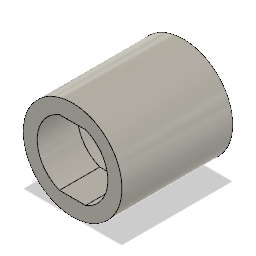
Nikon Labophot - Epifluorescence module adapter v3 (Autodesk Fusion 360 design; units mm, degrees)
Autodesk Fusion 360 part; units mm, degrees
note: some values were not read from the file. Set by a fixed rule: which sketch regions a step uses.
sketch "Sketch1" plane through (0, 0, 0) normal (0, 0, 1) x (1, 0, 0)
  circle A0 centre (0, 0) radius 22.5
  circle A1 centre (0, 0) radius 24.5
  dimension "d1" = 45
  dimension "d2" = 49
  measures "d1" diameter of A0
  measures "d2" diameter of A1
extrude "Extrude1" add sketch "Sketch1" against normal blind 35
sketch "Sketch2" plane through (0, 0, 0) normal (0, 0, 1) x (1, 0, 0)
  circle A0 centre (0, 0) radius 22.5
  circle A1 centre (0, 0) radius 24.5
  circle A2 centre (0, 0) radius 15
  circle A3 centre (0, 0) radius 17.5
  circle A4 centre (0, 0) radius 20
  line L0 (9.6825, 17.5) -> (-9.6825, 17.5)
  line L1 (-9.6825, -17.5) -> (9.6825, -17.5)
  line L2 (-11.6592, 16.25) -> (11.6592, 16.25)
  line L3 (-13.2288, 15) -> (13.2288, 15)
  line L4 (-13.2288, -15) -> (13.2288, -15)
  line L5 (-11.6592, -16.25) -> (11.6592, -16.25)
  dimension "d5" = 30
  dimension "d6" = 35
  dimension "d7" = 40
  dimension "d11" = 1.25
  dimension "d12" = 1.25
  measures "d5" diameter of A2
  measures "d6" diameter of A3
  measures "d7" diameter of A4
  measures "d11" distance of L2 L3
  measures "d12" distance of L4 L5
extrude "Extrude2" add sketch "Sketch2" along normal blind 20 contours A0 | A1 | A3 A4 L2 L3 | A3 A4 L3 L4 | A3 A4 L3 L4 | A3 A4 L2 L3 | A3 A4 L4 L5 | A3 A4 L4 L5 | A3 A4 L0 L2 | A3 L2 | A3 A4 L0 L2 | A3 L5 | A3 A4 L1 L5 | A3 A4 L1 L5 | A4 L0 | A4 L1
